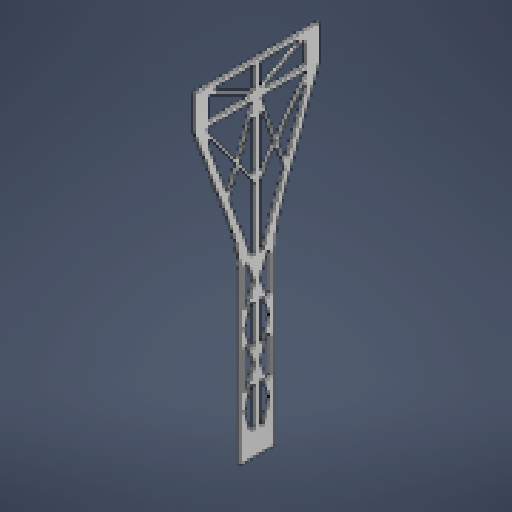
# Autodesk Inventor part: TUBE,CF,ARM
Saved by Autodesk Inventor 2024.3 (Build 283343000, 343)
## iProperties
Category: _
Manager: _
ILogicPurgeVersion: 0.0.0.0
OnSaveVersion: 3.5.0.0
OnSaveAssembly: COREAutomationManager
Created: 2025-03-06
Part Number: TUBE,CF,ARM
Checked By: 00
Engr Approved By: _
User Status: Work In Process
Material: Aluminum 3004-H32
Description: STANDARD (mm)
Document SubType Name: Sheet Metal
Mfg Approved By: John.Thibert
Designer: John.Thibert
Manufacturer: Standard
Standards Organization: Custom
Density: 2.71043 g/cm^3
Appearance: Aluminum - Polished
Sheet Metal Rule: Default
Mass: 169.09 g
Surface Area: 534.807 cm^2
Volume: 62.3849 cm^3
CN_MASS: 0.17
CN_SERVICEABLE: _
FIRST_DESCRIPTION: _
SECOND_DESCRIPTION: _
THIRD_DESCRIPTION: _
ModelCat: Uncategorized
MaterialName: Aluminum 3004-H32
Subject: _
Author: John.Thibert
Keywords: -
Revision Number: A
Autodesk Inventor part; units mm, degrees
ref_plane "YZ Plane" through (0, 0, 0) normal (1, 0, 0) x (0, 1, 0)
ref_plane "XZ Plane" through (0, 0, 0) normal (0, 1, 0) x (-1, 0, 0)
ref_plane "XY Plane" through (0, 0, 0) normal (0, 0, 1) x (1, 0, 0)
sketch "Sketch2" plane through (0, 0, 0) normal (1, 0, 0) x (0, 1, 0)
  line L0 (0, 88.9) -> (0, -88.9) construction
  line L1 (0, 88.9) -> (-25.4, 88.9)
  line L2 (-25.4, 88.9) -> (-174.6132, 34.5908)
  line L3 (0, 0) -> (-596.9, 0) construction
  arc A0 (-226.737, 25.4) -> (-174.6132, 34.5908) centre (-226.737, 177.8) ccw
  line L4 (-226.737, 25.4) -> (-469.9, 25.4)
  line L5 (-469.9, 25.4) -> (-469.9, 0)
  line L6 (0, 88.9) -> (25.4, 88.9)
  line L7 (25.4, 88.9) -> (25.4, -88.9)
  line L8 (25.4, -88.9) -> (0, -88.9)
  line L9 (0, -88.9) -> (-25.4, -88.9)
  line L10 (-25.4, -88.9) -> (-174.6132, -34.5908)
  arc A1 (-174.6132, -34.5908) -> (-226.737, -25.4) centre (-226.737, -177.8) ccw
  line L11 (-226.737, -25.4) -> (-469.9, -25.4)
  line L12 (-469.9, -25.4) -> (-469.9, 0)
  dimension "d6" = 177.8
  dimension "d7" = 596.9
  dimension "d8" = 152.4
  dimension "d9" = 70
  dimension "d10" = 50.8
  dimension "d11" = 25.4
  dimension "d12" = 127
  measures "d6" distance of L0.start L0.end
  measures "d7" distance of L3.start L3.end
  measures "d8" radius of A0
  measures "d9" angle of L0 L2
  measures "d10" diameter of L4 L3
  measures "d11" distance of L7.end L0.end
  measures "d12" distance from line of L3.end L5
extrude "Plate1" add sketch "Sketch2" along normal blind 3.175
sketch "Sketch3" plane through (3.175, 0, 0) normal (1, 0, 0) x (0, 0, -1)
  line L0 (-88.9, -25.4) -> (-88.9, 25.4) construction
  line L1 (-34.5908, -174.6132) -> (-88.9, -25.4) construction
  arc A0 (-25.4, -226.737) -> (-34.5908, -174.6132) centre (-177.8, -226.737) ccw construction
  line L2 (-25.4, -469.9) -> (-25.4, -226.737) construction
  line L3 (25.4, -469.9) -> (-25.4, -469.9) construction
  line L4 (25.4, -226.737) -> (25.4, -469.9) construction
  arc A1 (34.5908, -174.6132) -> (25.4, -226.737) centre (177.8, -226.737) ccw construction
  line L5 (88.9, -25.4) -> (34.5908, -174.6132) construction
  line L6 (88.9, 25.4) -> (88.9, -25.4) construction
  line L7 (-88.9, 25.4) -> (88.9, 25.4) construction
  line L8 (-3.175, 19.05) -> (-69.85, 19.05)
  line L9 (-69.85, 19.05) -> (-3.175, -15.4746)
  line L10 (-3.175, -15.4746) -> (-3.175, 19.05)
  line L11 (-248.92, 0) -> (248.92, 0) construction
  line L12 (0, -669.7491) -> (0, 141.2582) construction
  line L13 (-69.85, 15.4746) -> (-3.175, -19.05)
  line L14 (-3.175, -19.05) -> (-69.85, -19.05)
  line L15 (-69.85, -19.05) -> (-69.85, 15.4746)
  line L16 (-3.175, -233.0783) -> (-78.7637, -25.4)
  line L17 (-78.7637, -25.4) -> (-3.175, -25.4)
  line L18 (-3.175, -25.4) -> (-3.175, -233.0783)
  line L19 (-3.175, -25.4) -> (-40.9694, -129.2391) construction
  line L20 (-3.175, -30.0415) -> (-40.1247, -131.5599)
  line L21 (-4.8644, -25.4) -> (-41.814, -126.9184)
  line L22 (-78.7637, -25.4) -> (-29.4975, -93.0789)
  line L23 (-27.245, -96.1733) -> (-3.175, -129.2391)
  line L24 (-74.8366, -25.4) -> (-28.1884, -89.4823)
  line L25 (-25.9359, -92.5767) -> (-3.175, -123.8443)
  line L26 (-19.05, -208.0282) -> (-3.175, -251.6444)
  line L27 (-3.175, -251.6444) -> (-19.05, -295.2606)
  line L28 (-19.05, -295.2606) -> (-19.05, -208.0282)
  line L29 (-3.175, -260.9275) -> (-19.05, -304.5437)
  line L30 (-19.05, -304.5437) -> (-3.175, -348.1599)
  line L31 (-3.175, -348.1599) -> (-3.175, -260.9275)
  line L32 (-19.05, -310.8937) -> (-3.175, -354.5099)
  line L33 (-3.175, -363.793) -> (-19.05, -407.4092)
  line L34 (-19.05, -407.4092) -> (-3.175, -451.0254)
  line L35 (-3.175, -451.0254) -> (-3.175, -363.793)
  line L36 (-3.175, -354.5099) -> (-19.05, -398.1261)
  line L37 (-19.05, -398.1261) -> (-19.05, -310.8937)
  point P0 (0, 0)
  dimension "d14" = 19.05
  dimension "d15" = 6.35
  dimension "d16" = 3.175
  dimension "d17" = 38.1
  dimension "d18" = 6.35
  dimension "d19" = 9.525
  dimension "d20" = 6.35
  dimension "d21" = 1.5875
  dimension "d23" = 3.175
  dimension "d24" = 6.35
  dimension "d25" = 6.35
  dimension "d26" = 3.175
  dimension "d27" = 96.5155
  dimension "d30" = 102.8655
  constraints: 56 end point, 18 point on line, 8 parallel, 5 equal length, 3 collinear, 3 horizontal, 3 midpoint, 3 perpendicular, 2 vertical, 13 other
  measures "d14" distance from line of L0 L8.end
  measures "d15" distance between parallel lines of L7 L8
  measures "d16" distance between parallel lines of L13 L9
  measures "d17" distance between parallel lines of L14 L8
  measures "d18" diameter of L10 L12
  measures "d19" distance between parallel lines of L16 L1
  measures "d20" distance between parallel lines of L14 L17
  measures "d21" distance between parallel lines of L19 L20
  measures "d23" distance between parallel lines of L24 L22
  measures "d24" distance between parallel lines of L16 L26
  measures "d25" distance between parallel lines of L28 L2
  measures "d26" distance between parallel lines of L29 L27
  measures "d27" distance of L30.end L26.end
  measures "d30" distance of L26.end L32.end
extrude "Cut1" cut sketch "Sketch3" against normal blind 3.175 contours L10 L9 L8 | L13 L14 L15 | L16 L20 L23 L18 | L16 L22 L21 | L25 L20 L18 | L17 L21 L24 | L26 L27 L28 | L31 L30 L29 | L32 L36 L37 | L35 L34 L33
mirror "Mirror1" about plane through (0, 0, 0) normal (0, 0, 1) of "Cut1"
fillet "Corner Round1" radius 3.175 62 edges at (1.5875, -25.4, -74.8366) (1.5875, -89.4823, -28.1884) (1.5875, -25.4, -4.8644) (1.5875, 15.4746, -69.85) (1.5875, -19.05, -69.85) (1.5875, -19.05, -3.175) (1.5875, -92.5767, -25.9359) (1.5875, -123.8443, -3.175) (1.5875, -30.0415, -3.175) (1.5875, -304.5437, -19.05) (1.5875, -348.1599, -3.175) (1.5875, -260.9275, -3.175) (1.5875, -363.793, -3.175) (1.5875, -407.4092, -19.05) (1.5875, -451.0254, -3.175) (1.5875, -310.8937, -19.05) (1.5875, -398.1261, -19.05) (1.5875, -354.5099, -3.175) (1.5875, -208.0282, -19.05) (1.5875, -251.6444, -3.175) (1.5875, -295.2606, -19.05) (1.5875, -126.9184, -41.814) (1.5875, -93.0789, -29.4975) (1.5875, -25.4, -78.7637) (1.5875, -96.1733, -27.245) (1.5875, -131.5599, -40.1247) (1.5875, -129.2391, -3.175) (1.5875, -233.0783, -3.175) (1.5875, 19.05, -69.85) (1.5875, -15.4746, -3.175) (1.5875, 19.05, -3.175) (1.5875, -89.4823, 28.1884) (1.5875, -25.4, 74.8366) (1.5875, -25.4, 4.8644) (1.5875, -19.05, 69.85) (1.5875, 15.4746, 69.85) (1.5875, -19.05, 3.175) (1.5875, -123.8443, 3.175) (1.5875, -92.5767, 25.9359) (1.5875, -30.0415, 3.175) (1.5875, -348.1599, 3.175) (1.5875, -304.5437, 19.05) (1.5875, -260.9275, 3.175) (1.5875, -407.4092, 19.05) (1.5875, -363.793, 3.175) (1.5875, -451.0254, 3.175) (1.5875, -398.1261, 19.05) (1.5875, -354.5099, 3.175) (1.5875, -310.8937, 19.05) (1.5875, -295.2606, 19.05) (1.5875, -208.0282, 19.05) (1.5875, -251.6444, 3.175) (1.5875, -131.5599, 40.1247) (1.5875, -233.0783, 3.175) (1.5875, -96.1733, 27.245) (1.5875, -129.2391, 3.175) (1.5875, -15.4746, 3.175) (1.5875, 19.05, 3.175) (1.5875, 19.05, 69.85) (1.5875, -93.0789, 29.4975) (1.5875, -25.4, 78.7637) (1.5875, -126.9184, 41.814)
equation "\"d35\" = Thickness"
equation "\"d13\" = Thickness"
equation "\"BendRadius\" = 1.5 * Thickness"
equation "\"BendReliefWidth\" = Thickness"
equation "\"BendReliefDepth\" = 0.5 * Thickness"
equation "\"CornerReliefSize\" = 4 * Thickness"
equation "\"MinimumRemnant\" = 2 * Thickness"
equation "\"TransitionRadius\" = BendRadius"
equation "\"JacobiRadiusSize\" = BendRadius"
equation "\"GapSize\" = Thickness"
equation "\"Thickness\" = 3.175"
body "Solid2"
